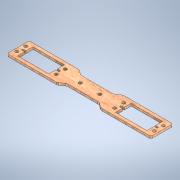
# Autodesk Inventor part: Brazo2Derecha
Saved by Autodesk Inventor 2022 (Build 260153000, 153)
## iProperties
Created: 2021-09-12
Part Number: Brazo2Derecha
Material: Wood (Birch)
Document SubType Name: Modeling
Designer: Administrador
Density: 0.55 g/cm^3
Appearance: Birch - Natural Polished
Author: Administrador
Autodesk Inventor part; units mm, degrees
ref_plane "YZ Plane" through (0, 0, 0) normal (1, 0, 0) x (0, 1, 0)
ref_plane "XZ Plane" through (0, 0, 0) normal (0, 1, 0) x (-1, 0, 0)
ref_plane "XY Plane" through (0, 0, 0) normal (0, 0, 1) x (1, 0, 0)
sketch "Sketch1" plane through (0, 0, 0) normal (0, 1, 0) x (-1, 0, 0)
  circle A0 centre (87, 18.3) radius 2
  line L0 (74.5, 9.3) -> (74.5, 27.3) construction
  line L1 (100.9626, 31.4151) -> (96.2822, 28.1849)
  line L2 (101.784, 5.06) -> (96.216, 8.54)
  line L3 (74.5, 9.3) -> (93.566, 9.3)
  line L4 (164, 4.3) -> (104.434, 4.3)
  line L5 (164, 32.3) -> (103.8026, 32.3)
  line L6 (74.5, 27.3) -> (93.4421, 27.3)
  line L7 (166, 30.3) -> (166, 6.3)
  line L8 (157, 28.3) -> (117, 28.3)
  line L9 (117, 8.3) -> (157, 8.3)
  circle A1 centre (62, 18.3) radius 2
  line L10 (48.0374, 31.4151) -> (52.7178, 28.1849)
  line L11 (47.216, 5.06) -> (52.784, 8.54)
  line L12 (74.5, 9.3) -> (55.434, 9.3)
  line L13 (-15, 4.3) -> (44.566, 4.3)
  line L14 (-15, 32.3) -> (45.1974, 32.3)
  line L15 (74.5, 27.3) -> (55.5579, 27.3)
  line L16 (-17, 30.3) -> (-17, 6.3)
  line L17 (-8, 28.3) -> (32, 28.3)
  line L18 (32, 8.3) -> (-8, 8.3)
  arc A2 (166, 30.3) -> (164, 32.3) centre (164, 30.3) ccw
  arc A3 (164, 4.3) -> (166, 6.3) centre (164, 6.3) ccw
  arc A4 (-17, 6.3) -> (-15, 4.3) centre (-15, 6.3) ccw
  arc A5 (-15, 32.3) -> (-17, 30.3) centre (-15, 30.3) ccw
  arc A6 (103.8026, 32.3) -> (100.9626, 31.4151) centre (103.8026, 27.3) ccw
  arc A7 (93.4421, 27.3) -> (96.2822, 28.1849) centre (93.4421, 32.3) ccw
  arc A8 (101.784, 5.06) -> (104.434, 4.3) centre (104.434, 9.3) ccw
  arc A9 (96.216, 8.54) -> (93.566, 9.3) centre (93.566, 4.3) ccw
  arc A10 (55.434, 9.3) -> (52.784, 8.54) centre (55.434, 4.3) ccw
  arc A11 (44.566, 4.3) -> (47.216, 5.06) centre (44.566, 9.3) ccw
  arc A12 (52.7178, 28.1849) -> (55.5579, 27.3) centre (55.5579, 32.3) ccw
  arc A13 (48.0374, 31.4151) -> (45.1974, 32.3) centre (45.1974, 27.3) ccw
  arc A14 (39, 25.3) -> (39, 22.8) centre (37.2507, 24.05) ccw projected
  arc A15 (39, 13.8) -> (39, 11.3) centre (37.2507, 12.55) ccw projected
  arc A16 (-15, 11.3) -> (-15, 13.8) centre (-13.2507, 12.55) ccw projected
  arc A17 (-15, 22.8) -> (-15, 25.3) centre (-13.2507, 24.05) ccw projected
  arc A18 (110, 22.8) -> (110, 25.3) centre (111.7493, 24.05) ccw projected
  arc A19 (110, 11.3) -> (110, 13.8) centre (111.7493, 12.55) ccw projected
  arc A20 (164, 13.8) -> (164, 11.3) centre (162.2507, 12.55) ccw projected
  arc A21 (164, 25.3) -> (164, 22.8) centre (162.2507, 24.05) ccw projected
  circle A22 centre (162.2507, 24.05) radius 1.95
  circle A23 centre (162.2507, 12.55) radius 1.95
  circle A24 centre (111.7493, 24.05) radius 1.95
  circle A25 centre (111.7493, 12.55) radius 1.95
  circle A26 centre (37.2507, 24.05) radius 1.95
  circle A27 centre (37.2507, 12.55) radius 1.95
  circle A28 centre (-13.2507, 24.05) radius 1.95
  circle A29 centre (-13.2507, 12.55) radius 1.95
  circle A30 centre (22, 18.3) radius 4.375 projected
  circle A31 centre (147, 18.3) radius 1.3 projected
  circle A32 centre (147, 18.3) radius 1.3 projected
  line L19 (32, 28.3) -> (32, 19.3)
  line L20 (32, 19.3) -> (36, 19.3)
  line L21 (36, 19.3) -> (36, 17.3)
  line L22 (36, 17.3) -> (32, 17.3)
  line L23 (32, 17.3) -> (32, 8.3)
  line L24 (-8, 28.3) -> (-8, 19.3)
  line L25 (-8, 19.3) -> (-12, 19.3)
  line L26 (-12, 19.3) -> (-12, 17.3)
  line L27 (-12, 17.3) -> (-8, 17.3)
  line L28 (-8, 17.3) -> (-8, 8.3)
  line L29 (117, 28.3) -> (117, 19.3)
  line L30 (117, 19.3) -> (113, 19.3)
  line L31 (113, 19.3) -> (113, 17.3)
  line L32 (113, 17.3) -> (117, 17.3)
  line L33 (117, 17.3) -> (117, 8.3)
  line L34 (157, 8.3) -> (157, 17.3)
  line L35 (157, 17.3) -> (161, 17.3)
  line L36 (161, 17.3) -> (161, 19.3)
  line L37 (161, 19.3) -> (157, 19.3)
  line L38 (157, 19.3) -> (157, 28.3)
  point P0 (166, 4.3)
  point P1 (166, 32.3)
  point P2 (1.5, 26.1095)
  point P3 (22.5, 26.1095)
  point P4 (95, 27.3)
  point P5 (95, 9.3)
  point P6 (102.2448, 32.3)
  point P7 (103, 4.3)
  point P8 (-17, 4.3)
  point P9 (-17, 32.3)
  point P10 (54, 27.3)
  point P11 (54, 9.3)
  point P12 (46.7552, 32.3)
  point P13 (46, 4.3)
  dimension "d19" = 12.5
  dimension "d20" = 9
  dimension "d21" = 9
  dimension "d22" = 14
  dimension "d23" = 14
  dimension "d25" = 5
  dimension "d26" = 91.5
  dimension "d29" = 40
  dimension "d30" = 20
  dimension "d31" = 4
  dimension "d35" = 2
  dimension "d36" = 5
  dimension "d37" = 5
  dimension "d38" = 5
  dimension "d39" = 5
  dimension "d40" = 5
  dimension "d41" = 5
  dimension "d42" = 5
  dimension "d43" = 5
  dimension "d44" = 3.9
  dimension "d45" = 3.9
  dimension "d46" = 3.9
  dimension "d47" = 3.9
  dimension "d48" = 3.9
  dimension "d49" = 3.9
  dimension "d50" = 3.9
  dimension "d51" = 3.9
  dimension "d52" = 125
  dimension "d53" = 40
  dimension "d54" = 9
  dimension "d55" = 4
  dimension "d56" = 2
  dimension "d57" = 4
  dimension "d58" = 9
  dimension "d59" = 4
  dimension "d60" = 2
  dimension "d61" = 4
  dimension "d62" = 9
  dimension "d63" = 9
  dimension "d64" = 4
  dimension "d65" = 2
  dimension "d66" = 4
  dimension "d67" = 9
  dimension "d68" = 9
  dimension "d69" = 4
  dimension "d70" = 2
  dimension "d71" = 4
  dimension "d72" = 9
  dimension "d73" = 25
  constraints: 78 end point, 28 point on line, 24 point on circle, 24 tangent, 22 centre point, 11 symmetric about line, 10 perpendicular, 8 coincident, 5 vertical, 3 equal radius, 2 horizontal, 1 parallel, 1 other
  measures "d19" distance from line of L0 A0.centre
  measures "d20" distance from line of L6 A0.centre
  measures "d21" distance from line of L3 A0.centre
  measures "d22" distance from line of L4 A0.centre
  measures "d23" distance from line of L5 A0.centre
  measures "d25" distance between parallel lines of L3 L4
  measures "d26" distance between parallel lines of L0 L7
  measures "d29" distance of L9.end L9.start
  measures "d30" distance of L9.start L8.end
  measures "d31" distance between parallel lines of L5 L8
  measures "d35" radius of A2
  measures "d36" radius of A6
  measures "d37" radius of A7
  measures "d38" radius of A8
  measures "d39" radius of A9
  measures "d40" radius of A10
  measures "d41" radius of A11
  measures "d42" radius of A12
  measures "d43" radius of A13
  measures "d44" diameter of A22
  measures "d45" diameter of A23
  measures "d46" diameter of A24
  measures "d47" diameter of A25
  measures "d48" diameter of A26
  measures "d49" diameter of A27
  measures "d50" diameter of A28
  measures "d51" diameter of A29
  measures "d52" distance of A31.centre A30.centre
  measures "d53" distance of A1.centre A30.centre
  measures "d54" distance of L17.end L19.end
  measures "d55" distance of L19.end L20.end
  measures "d56" distance of L20.end L21.end
  measures "d57" distance of L21.end L22.end
  measures "d58" distance of L17.start L24.end
  measures "d59" distance of L24.end L25.end
  measures "d60" distance of L25.end L26.end
  measures "d61" distance of L26.end L27.end
  measures "d62" distance of L27.end L18.end
  measures "d63" distance of L8.end L29.end
  measures "d64" distance of L29.end L30.end
  measures "d65" distance of L30.end L31.end
  measures "d66" distance of L31.end L32.end
  measures "d67" distance of L32.end L9.start
  measures "d68" distance of L9.end L34.end
  measures "d69" distance of L34.end L35.end
  measures "d70" distance of L35.end L36.end
  measures "d71" distance of L36.end L37.end
  measures "d72" distance of L37.end L8.start
  measures "d73" distance of A0.centre A1.centre
extrude "Extrusion1" add sketch "Sketch1" along normal blind 3 contours A6 L5 A2 L7 A3 L4 A8 L2 A9 L3 L12 A10 L11 A11 L13 A4 L16 A5 L14 A13 L10 A12 L15 L6 A7 L1
body "Solid1"
